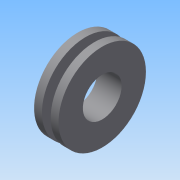
# Autodesk Inventor part: держатель  бабины
Saved by Autodesk Inventor 2017 (Build 210142000, 142)
## iProperties
Part Number: держатель  бабины
Material: Типовые
Document SubType Name: Modeling
Designer: Max
Mass: 4.06271 g
Surface Area: 35.1532 cm^2
Volume: 4.06271 cm^3
Density: 1 g/cm^3
Appearance: Резина — синяя
Author: Max
Autodesk Inventor part; units mm, degrees
ref_plane "YZ Plane" through (0, 0, 0) normal (1, 0, 0) x (0, 1, 0)
ref_plane "XZ Plane" through (0, 0, 0) normal (0, 1, 0) x (-1, 0, 0)
ref_plane "XY Plane" through (0, 0, 0) normal (0, 0, 1) x (1, 0, 0)
sketch "Эскиз1" plane through (0, 0, 0) normal (1, 0, 0) x (0, 1, 0)
  circle A0 centre (0, 0) radius 11.1
  circle A1 centre (0, 0) radius 17.5
  circle A2 centre (0, 0) radius 14.1
  dimension "d0" = 22.2
  dimension "d1" = 35
  dimension "d2" = 3
  dimension "d3" = 3.4
  constraints: 3 centre point, 3 coincident
  measures "d0" diameter of A0
  measures "d1" diameter of A1
  measures "d2" radial gap between concentric circles of A0 A2
  measures "d3" radial gap between concentric circles of A2 A1
extrude "Выдавливание1" add sketch "Эскиз1" along normal mid plane 10 contours A1 | A2
extrude "Выдавливание2" cut sketch "Эскиз1" along normal mid plane 5 contours A1
